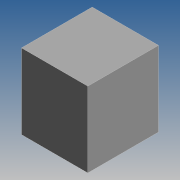
# Autodesk Inventor part: 2usb
Saved by Autodesk Inventor 2017 (Build 210142000, 142)
## iProperties
Created: 2018-10-05
Part Number: 2usb
Material: Générique
Document SubType Name: Modeling
Designer: Gilles Mottiez
Density: 1 g/cm^3
Appearance: Par défaut
Author: Gilles Mottiez
Autodesk Inventor part; units mm, degrees
ref_plane "YZ Plane" through (0, 0, 0) normal (1, 0, 0) x (0, 1, 0)
ref_plane "XZ Plane" through (0, 0, 0) normal (0, 1, 0) x (-1, 0, 0)
ref_plane "XY Plane" through (0, 0, 0) normal (0, 0, 1) x (1, 0, 0)
sketch "Sketch1" plane through (0, 0, 0) normal (0, 0, 1) x (1, 0, 0)
  line L0 (0, 0) -> (15, 0)
  line L1 (15, 0) -> (15, 16)
  line L2 (15, 16) -> (0, 16)
  line L3 (0, 16) -> (0, 0)
  dimension "d0" = 15
  dimension "d1" = 16
  constraints: 8 end point, 2 parallel, 1 horizontal, 1 perpendicular
  measures "d0" distance of L2.end L1.end
  measures "d1" distance of L1.end L0.end
extrude "Extrusion1" add sketch "Sketch1" along normal blind 17
sketch "Esquisse2" plane through (0, 0, 0) normal (0, 0, -1) x (-1, 0, 0)
  line L0 (0, 0) -> (-15, 0) construction
  line L1 (0, 16) -> (0, 0) construction
  line L2 (-15, 16) -> (0, 16) construction
  line L3 (-15, 0) -> (-15, 16) construction
  line L4 (-13.5, 15) -> (-1.5, 15)
  line L5 (-1.5, 15) -> (-1.5, 10)
  line L6 (-1.5, 10) -> (-13.5, 10)
  line L7 (-13.5, 10) -> (-13.5, 15)
  line L8 (-13.5, 6) -> (-1.5, 6)
  line L9 (-1.5, 6) -> (-1.5, 1)
  line L10 (-1.5, 1) -> (-13.5, 1)
  line L11 (-13.5, 1) -> (-13.5, 6)
  line L12 (-7.5, 0) -> (-7.5, 16) construction
  dimension "d4" = 12
  dimension "d5" = 5
  dimension "d6" = 5
  dimension "d7" = 1
  dimension "d8" = 4
  constraints: 18 end point, 4 parallel, 2 horizontal, 2 midpoint, 2 perpendicular, 2 point on line, 1 vertical alignment, 1 other
  measures "d4" distance of L4.start L4.end
  measures "d5" distance of L4.end L5.end
  measures "d6" distance of L8.end L9.end
  measures "d7" distance between parallel lines of L0 L10
  measures "d8" distance between parallel lines of L8 L6
extrude "Extrusion2" cut sketch "Esquisse2" against normal blind 15
